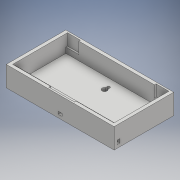
# Autodesk Inventor part: housing
Saved by Autodesk Inventor 2018.1 (Build 221171000, 171)
## iProperties
Created: 2018-03-22
Part Number: housing
Material: Generic
Document SubType Name: Modeling
Designer: wharr
Density: 1 g/cm^3
Appearance: Default
Author: wharr
Autodesk Inventor part; units mm, degrees
ref_plane "YZ Plane" through (0, 0, 0) normal (1, 0, 0) x (0, 1, 0)
ref_plane "XZ Plane" through (0, 0, 0) normal (0, 1, 0) x (-1, 0, 0)
ref_plane "XY Plane" through (0, 0, 0) normal (0, 0, 1) x (1, 0, 0)
sketch "Sketch1" plane through (0, 0, 0) normal (0, 0, 1) x (1, 0, 0)
  line L0 (-100, -52.5) -> (100, -52.5)
  line L1 (100, -52.5) -> (100, 52.5)
  line L2 (100, 52.5) -> (-100, 52.5)
  line L3 (-100, 52.5) -> (-100, -52.5)
  line L4 (-100, -52.5) -> (100, 52.5) construction
  line L5 (100, -52.5) -> (-100, 52.5) construction
  line L6 (-106.35, 58.85) -> (106.35, 58.85)
  line L7 (106.35, 58.85) -> (106.35, -58.85)
  line L8 (106.35, -58.85) -> (-106.35, -58.85)
  line L9 (-106.35, -58.85) -> (-106.35, 58.85)
  point P0 (0, 0)
  dimension "d0" = 200
  dimension "d1" = 105
  dimension "d2" = 6.35
  constraints: 20 end point, 4 parallel, 2 midpoint, 2 perpendicular, 1 horizontal, 3 other
  measures "d0" distance of L1.end L2.end
  measures "d1" distance of L0.end L1.end
  measures "d2" distance between parallel lines of L2 L6
extrude "Extrusion1" add sketch "Sketch1" against normal blind 40
sketch "Sketch2" plane through (-100, 52.5, 0) normal (0, -1, 0) x (1, 0, 0)
  line L0 (200, -40) -> (0, -40) projected
  line L1 (0, 0) -> (0, -40) projected
  line L2 (200, -40) -> (0, -40)
  line L3 (0, -40) -> (0, -33.65)
  line L4 (0, -33.65) -> (200, -33.65)
  line L5 (200, -33.65) -> (200, -40)
  point P0 (100, 0)
  dimension "d5" = 6.35
  constraints: 8 end point, 2 parallel, 1 horizontal, 1 perpendicular, 1 point on line
  measures "d5" distance between parallel lines of L0 L4
extrude "Extrusion2" add sketch "Sketch2" along normal up to next
sketch "Sketch4" plane through (0, 0, -40) normal (0, 0, -1) x (-1, 0, 0)
  line L0 (106.35, 58.85) -> (-106.35, 58.85) projected
  line L1 (0, 58.85) -> (0, -58.85)
  line L2 (-106.35, -58.85) -> (106.35, -58.85) projected
  arc A0 (-2.5, 33.1801) -> (2.5, 33.1801) centre (0, 28.85) ccw
  line L3 (0, 28.85) -> (0, 36.85) construction
  line L4 (2.5, 33.1801) -> (2.5, 36.85)
  line L5 (-2.5, 36.85) -> (-2.5, 33.1801)
  arc A1 (2.5, 36.85) -> (-2.5, 36.85) centre (0, 36.85) ccw
  point P0 (0, 0)
  point P1 (0, 32.85)
  dimension "d14" = 10
  dimension "d15" = 5
  dimension "d17" = 30
  dimension "d18" = 8
  constraints: 10 end point, 4 point on circle, 3 midpoint, 2 centre point, 2 point on line, 2 tangent, 1 parallel
  measures "d14" diameter of A0
  measures "d15" diameter of A1
  measures "d17" distance from line of L3.start L0
  measures "d18" distance of L3.end L3.start
extrude "Extrusion4" cut sketch "Sketch4" against normal through all
sketch "Sketch5" plane through (100, -52.5, 0) normal (-1, 0, 0) x (0, 0, 1)
  line L0 (-33.65, 105) -> (-33.65, 0) projected
  line L1 (0, 0) -> (-33.65, 0) projected
  line L2 (-33.65, 0) -> (-26.15, 0)
  line L3 (-26.15, 0) -> (-26.15, 5)
  line L4 (-26.15, 5) -> (-33.65, 5)
  line L5 (-33.65, 5) -> (-33.65, 0)
  point P0 (0, 52.5)
  dimension "d21" = 7.5
  dimension "d22" = 5
  constraints: 8 end point, 2 parallel, 1 horizontal, 1 perpendicular
  measures "d21" distance of L4.end L3.end
  measures "d22" distance of L3.end L2.end
extrude "Extrusion5" cut sketch "Sketch5" against normal through all
sketch "Sketch6" plane through (-100, -52.5, 0) normal (1, 0, 0) x (0, 0, -1)
  line L0 (0, 0) -> (33.65, 0) projected
  line L1 (0, 0) -> (0, 105) projected
  line L2 (0, 105) -> (33.65, 105) projected
  line L3 (2.5, 0) -> (5.5, 0)
  line L4 (5.5, 0) -> (5.5, 3)
  line L5 (5.5, 3) -> (2.5, 3)
  line L6 (2.5, 3) -> (2.5, 0)
  point P0 (0, 52.5)
  dimension "d26" = 2.5
  dimension "d27" = 3
  dimension "d28" = 3
  constraints: 8 end point, 2 parallel, 1 horizontal, 1 perpendicular, 1 point on line
  measures "d26" distance between parallel lines of L1 L6
  measures "d27" distance of L3.end L4.end
  measures "d28" distance of L4.end L5.end
extrude "Extrusion6" add sketch "Sketch6" along normal up to next
sketch "Sketch7" plane through (0, 0, 0) normal (0, 0, 1) x (1, 0, 0)
  line L0 (106.35, -58.85) -> (-106.35, -58.85) projected
  line L1 (0, -58.85) -> (0, -52.5)
  line L2 (-100, -52.5) -> (106.35, -52.5) projected
  line L3 (-25.4, -55.675) -> (25.4, -55.675)
  line L4 (25.4, -55.675) -> (25.4, -52.5)
  line L5 (25.4, -52.5) -> (-25.4, -52.5)
  line L6 (-25.4, -52.5) -> (-25.4, -55.675)
  line L7 (-25.4, -55.675) -> (25.4, -52.5) construction
  line L8 (25.4, -55.675) -> (-25.4, -52.5) construction
  arc A0 (25.4, -55.675) -> (28.575, -52.5) centre (25.4, -52.5) ccw construction
  arc A1 (-28.575, -52.5) -> (-25.4, -55.675) centre (-25.4, -52.5) ccw construction
  point P0 (0, 0)
  point P1 (0, -54.0875)
  dimension "d32" = 50.8
  dimension "d33" = 3.175
  constraints: 14 end point, 4 point on circle, 4 point on line, 3 midpoint, 2 centre point, 2 parallel, 2 symmetric about line, 1 coincident, 1 horizontal, 1 perpendicular, 1 vertical, 1 other
  measures "d32" distance of L3.start L3.end
  measures "d33" radius of A0
extrude "Extrusion7" cut sketch "Sketch7" against normal up to surface (2.5 mm away)
sketch "Sketch8" plane through (0, 0, 0) normal (0, 0, 1) x (1, 0, 0)
  line L0 (-100, -52.5) -> (-100, 52.5) projected
  line L1 (-100, 52.5) -> (-74.6, 52.5)
  line L2 (-74.6, 52.5) -> (-74.6, 55.675)
  line L3 (-74.6, 55.675) -> (-100, 55.675)
  line L4 (-100, 55.675) -> (-100, 52.5)
  point P0 (0, 0)
  dimension "d36" = 25.4
  dimension "d37" = 3.175
  constraints: 8 end point, 2 parallel, 1 horizontal, 1 perpendicular
  measures "d36" distance of L3.end L2.end
  measures "d37" distance of L1.end L2.end
extrude "Extrusion8" cut sketch "Sketch8" against normal blind 22.86
mirror "Mirror1" about plane through (0, 0, 0) normal (1, 0, 0) of "Extrusion8"
sketch "Sketch9" plane through (-100, -52.5, -33.65) normal (0, 1, 0) x (1, 0, 0)
  line L0 (0, 0) -> (206.35, 0) projected
  line L1 (96.2535, -5.0038) -> (103.7465, -5.0038)
  line L2 (103.7465, -5.0038) -> (103.7465, 0)
  line L3 (103.7465, 0) -> (96.2535, 0)
  line L4 (96.2535, 0) -> (96.2535, -5.0038)
  line L5 (206.35, 6.35) -> (-6.35, 6.35) projected
  line L6 (100, 6.35) -> (100, -33.65)
  line L7 (125.4, -33.65) -> (74.6, -33.65) projected
  point P0 (100, 0)
  dimension "d40" = 7.493
  dimension "d41" = 5.0038
  constraints: 10 end point, 2 midpoint, 2 parallel, 2 perpendicular, 1 collinear, 1 horizontal, 1 point on line
  measures "d40" distance of L3.end L2.end
  measures "d41" distance of L2.end L1.end
extrude "Extrusion9" cut sketch "Sketch9" against normal through all
body "Solid1"
